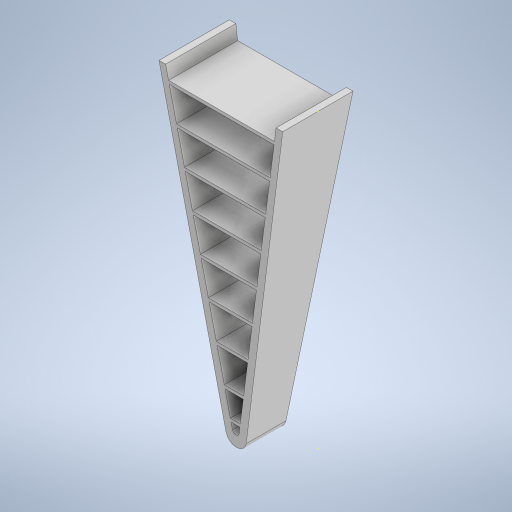
# Autodesk Inventor part: finley_gripper
Saved by Autodesk Inventor 2024 (Build 280153000, 153)
## iProperties
Created: 2024-09-21
Part Number: finley_gripper
Material: 一般
Document SubType Name: Modeling
Designer: 1412z
Density: 1 g/cm^3
Appearance: 既定
Author: 1412z
Autodesk Inventor part; units mm, degrees
ref_plane "YZ Plane" through (0, 0, 0) normal (1, 0, 0) x (0, 1, 0)
ref_plane "XZ Plane" through (0, 0, 0) normal (0, 1, 0) x (-1, 0, 0)
ref_plane "XY Plane" through (0, 0, 0) normal (0, 0, 1) x (1, 0, 0)
sketch "スケッチ1" plane through (0, 0, 0) normal (0, 0, 1) x (1, 0, 0)
  line L0 (0, 0) -> (-37.5, 0)
  line L1 (-18.75, -110) -> (0, 0)
  line L2 (-18.75, -110) -> (-37.5, 0)
  dimension "d0" = 37.5
  constraints: 6 end point, 1 horizontal
  measures "d0" distance of L0.start L0.end
extrude "押し出し1" add sketch "スケッチ1" along normal mid plane 21.3
sketch "スケッチ2" plane through (0, 0, 10.65) normal (0, 0, 1) x (1, 0, 0)
  line L0 (0, 0) -> (-37.5, 0) projected
  line L1 (-2, 0) -> (-35.5, 0)
  line L2 (-35.5, 0) -> (-18.75, -96.0642)
  line L3 (-18.75, -96.0642) -> (-2, 0)
  dimension "d4" = 33.5
  constraints: 6 end point, 2 point on line
  measures "d4" distance of L1.start L1.end
extrude "押し出し2" cut sketch "スケッチ2" against normal blind 21.3
fillet "フィレット3" [suppressed]
fillet "フィレット4" radius 1 1 edges at (-18.75, -96.0642, 0)
fillet "フィレット5" radius 3.1 1 edges at (-18.75, -110, 0)
sketch "スケッチ3" plane through (0, 0, 10.65) normal (0, 0, 1) x (1, 0, 0)
  line L0 (-2, 0) -> (-17.7649, -90.4143) projected
  line L1 (-2.6975, -4) -> (-34.8025, -4)
  line L2 (-19.7351, -90.4143) -> (-35.5, 0) projected
  line L3 (-2.6975, -4) -> (-2.6975, -5)
  line L4 (-2.6975, -5) -> (-34.8025, -5)
  line L5 (-34.8025, -5) -> (-34.8025, -4)
  point P0 (0, 0)
  dimension "d11" = 1
  constraints: 8 end point, 2 perpendicular, 2 point on line, 1 horizontal, 1 parallel
  measures "d11" distance of L1.start L3.end
extrude "押し出し3" add sketch "スケッチ3" against normal blind 21.3
sketch "スケッチ4" plane through (0, 0, 10.65) normal (0, 0, 1) x (1, 0, 0)
  line L0 (-3.8318, -14.75) -> (-33.6682, -14.75)
  line L1 (-33.6682, -14.75) -> (-33.6682, -15.75)
  line L2 (-33.6682, -15.75) -> (-3.8318, -15.75)
  line L3 (-3.8318, -15.75) -> (-3.8318, -14.75)
  line L4 (-3.8318, -14.75) -> (-33.6682, -15.75) construction
  line L5 (-33.6682, -14.75) -> (-3.8318, -15.75) construction
  line L6 (-5.8662, -25.5) -> (-31.6338, -25.5)
  line L7 (-31.6338, -25.5) -> (-31.6338, -26.5)
  line L8 (-31.6338, -26.5) -> (-5.8662, -26.5)
  line L9 (-5.8662, -26.5) -> (-5.8662, -25.5)
  line L10 (-5.8662, -25.5) -> (-31.6338, -26.5) construction
  line L11 (-31.6338, -25.5) -> (-5.8662, -26.5) construction
  line L12 (-6.9432, -36.25) -> (-30.5568, -36.25)
  line L13 (-30.5568, -36.25) -> (-30.5568, -37.25)
  line L14 (-30.5568, -37.25) -> (-6.9432, -37.25)
  line L15 (-6.9432, -37.25) -> (-6.9432, -36.25)
  line L16 (-6.9432, -36.25) -> (-30.5568, -37.25) construction
  line L17 (-30.5568, -36.25) -> (-6.9432, -37.25) construction
  line L18 (-9.5162, -47) -> (-27.9838, -47)
  line L19 (-27.9838, -47) -> (-27.9838, -48)
  line L20 (-27.9838, -48) -> (-9.5162, -48)
  line L21 (-9.5162, -48) -> (-9.5162, -47)
  line L22 (-9.5162, -47) -> (-27.9838, -48) construction
  line L23 (-27.9838, -47) -> (-9.5162, -48) construction
  line L24 (-11.1317, -57.75) -> (-26.3683, -57.75)
  line L25 (-26.3683, -57.75) -> (-26.3683, -58.75)
  line L26 (-26.3683, -58.75) -> (-11.1317, -58.75)
  line L27 (-11.1317, -58.75) -> (-11.1317, -57.75)
  line L28 (-11.1317, -57.75) -> (-26.3683, -58.75) construction
  line L29 (-26.3683, -57.75) -> (-11.1317, -58.75) construction
  line L30 (-12.8071, -68.5) -> (-24.6929, -68.5)
  line L31 (-24.6929, -68.5) -> (-24.6929, -69.5)
  line L32 (-24.6929, -69.5) -> (-12.8071, -69.5)
  line L33 (-12.8071, -69.5) -> (-12.8071, -68.5)
  line L34 (-12.8071, -68.5) -> (-24.6929, -69.5) construction
  line L35 (-24.6929, -68.5) -> (-12.8071, -69.5) construction
  line L36 (-14.557, -80.25) -> (-22.943, -80.25)
  line L37 (-22.943, -80.25) -> (-22.943, -79.25)
  line L38 (-22.943, -79.25) -> (-14.557, -79.25)
  line L39 (-14.557, -79.25) -> (-14.557, -80.25)
  line L40 (-14.557, -80.25) -> (-22.943, -79.25) construction
  line L41 (-22.943, -80.25) -> (-14.557, -79.25) construction
  line L42 (-16.5299, -87.5) -> (-20.9701, -87.5)
  line L43 (-20.9701, -87.5) -> (-20.9701, -88.5)
  line L44 (-20.9701, -88.5) -> (-16.5299, -88.5)
  line L45 (-16.5299, -88.5) -> (-16.5299, -87.5)
  line L46 (-16.5299, -87.5) -> (-20.9701, -88.5) construction
  line L47 (-20.9701, -87.5) -> (-16.5299, -88.5) construction
  point P0 (0, 0)
  point P1 (-18.75, -15.25)
  point P2 (-18.75, -26)
  point P3 (-18.75, -36.75)
  point P4 (-18.75, -47.5)
  point P5 (-18.75, -58.25)
  point P6 (-18.75, -69)
  point P7 (-18.75, -79.75)
  point P8 (-18.75, -88)
  dimension "d14" = 1
  dimension "d15" = 1
  dimension "d16" = 1
  dimension "d17" = 1
  dimension "d18" = 1
  dimension "d19" = 1
  dimension "d20" = 1
  dimension "d21" = 1
  constraints: 96 end point, 16 midpoint, 16 parallel, 8 horizontal, 8 perpendicular
  measures "d14" distance of L1.end L0.end
  measures "d15" distance of L7.end L6.end
  measures "d16" distance of L13.end L12.end
  measures "d17" distance of L19.end L18.end
  measures "d18" distance of L25.end L24.end
  measures "d19" distance of L31.end L30.end
  measures "d20" distance of L36.end L37.end
  measures "d21" distance of L43.end L42.end
extrude "押し出し4" add sketch "スケッチ4" against normal blind 21.3
sketch "スケッチ5" plane through (-20.0689, -88.5, 10.65) normal (0, -1, 0) x (1, 0, 0)
  point P0 (20.0689, -10.65)
sketch "スケッチ6" plane through (0, 0, 0) normal (0, 0, 1) x (1, 0, 0)
  point P0 (0, 0)
sketch "スケッチ7" plane through (0, 0, 0) normal (1, 0, 0) x (0, 1, 0)
  line L0 (-94.651, -10.65) -> (-94.651, 10.65) projected
  line L1 (-94.651, 0) -> (-94.651, 5.9)
  line L2 (-94.651, 0) -> (-94.651, -5.9)
  line L3 (0, 10.65) -> (-4, 10.65) projected
  line L4 (-94.651, 5.9) -> (0, 10.65)
  line L5 (0, 10.65) -> (-94.651, 10.65)
  line L6 (-80.25, 10.65) -> (-87.5, 10.65) projected
  line L7 (-94.651, 5.9) -> (-94.651, 10.65)
  line L8 (0, -10.65) -> (-92.0719, -10.65) projected
  line L9 (-94.651, -5.9) -> (0, -10.65)
  line L10 (-92.0719, -10.65) -> (-94.651, -10.65) projected
  line L11 (0, -10.65) -> (-94.651, -10.65)
  line L12 (-94.651, -10.65) -> (-94.651, -5.9)
  point P0 (0, 0)
  dimension "d24" = 5.9
  dimension "d25" = 5.9
  constraints: 16 end point, 4 collinear, 2 point on line, 1 midpoint
  measures "d24" distance of L1.start L1.end
  measures "d25" distance of L1.start L2.end
extrude "押し出し5" cut sketch "スケッチ7" along normal mid plane 100
